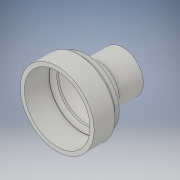
# Autodesk Inventor part: adapter
Saved by Autodesk Inventor 2019 (Build 230136000, 136)
## iProperties
Created: 2020-03-31
Part Number: adapter
Material: Generic
Document SubType Name: Modeling
Designer: Bishoy
Density: 1 g/cm^3
Appearance: Default
Author: Bishoy
Autodesk Inventor part; units mm, degrees
ref_plane "YZ Plane" through (0, 0, 0) normal (1, 0, 0) x (0, 1, 0)
ref_plane "XZ Plane" through (0, 0, 0) normal (0, 1, 0) x (-1, 0, 0)
ref_plane "XY Plane" through (0, 0, 0) normal (0, 0, 1) x (1, 0, 0)
sketch "Sketch1" plane through (0, 0, 0) normal (0, 0, 1) x (1, 0, 0)
  circle A0 centre (0, 0) radius 20
  circle A1 centre (0, 0) radius 22.5
  dimension "d0" = 40
  dimension "d1" = 45
  constraints: 2 centre point, 2 coincident
  measures "d0" diameter of A0
  measures "d1" diameter of A1
extrude "Extrusion1" add sketch "Sketch1" along normal blind 15
extrude "Extrusion2" add sketch "Sketch1" against normal blind 10 contours A0
sketch "Sketch2" plane through (0, 0, -10) normal (0, 0, -1) x (-1, 0, 0)
  circle A0 centre (0, 0) radius 12.5
  circle A1 centre (0, 0) radius 10
  dimension "d6" = 25
  dimension "d7" = 20
  constraints: 2 centre point, 2 coincident
  measures "d6" diameter of A0
  measures "d7" diameter of A1
extrude "Extrusion3" add sketch "Sketch2" along normal blind 15
chamfer "Chamfer1" distance 7.25 angle 45 1 edges at (-20, 0, -10)
chamfer "Chamfer2" distance 2.25 angle 45 1 edges at (-22.5, 0, 0)
extrude "Extrusion4" cut sketch "Sketch2" against normal blind 15 contours A1
sketch "Sketch3" plane through (0, 0, 0) normal (0, 0, 1) x (1, 0, 0)
  circle A0 centre (0, 0) radius 17.5
  dimension "d18" = 35
  constraints: 1 centre point, 1 coincident
  measures "d18" diameter of A0
extrude "Extrusion5" cut sketch "Sketch3" against normal blind 3.5
chamfer "Chamfer3" distance 7.5 angle 45 1 edges at (10, 0, -3.5)
chamfer "Chamfer4" distance 2.25 angle 45 1 edges at (-17.5, 0, 0)
body "Solid1"
